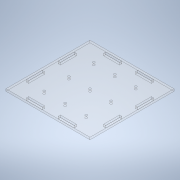
# Autodesk Inventor part: Box top
Saved by Autodesk Inventor 2021 (Build 250183000, 183)
## iProperties
Created: 2019-12-19
Part Number: Box top
Material: PMMA Plastic
Document SubType Name: Modeling
Designer: jstr255
Density: 1.188 g/cm^3
Appearance: Polycarbonate - Clear
Mass: 42.6667 g
Surface Area: 267.032 cm^2
Volume: 35.9147 cm^3
Author: jstr255
Autodesk Inventor part; units mm, degrees
ref_plane "YZ Plane" through (0, 0, 0) normal (1, 0, 0) x (0, 1, 0)
ref_plane "XZ Plane" through (0, 0, 0) normal (0, 1, 0) x (-1, 0, 0)
ref_plane "XY Plane" through (0, 0, 0) normal (0, 0, 1) x (1, 0, 0)
sketch "Sketch1" plane through (0, 0, 0) normal (0, 1, 0) x (-1, 0, 0)
  line L0 (21.2, 0) -> (21.2, -3)
  line L1 (42.4, 0) -> (42.4, -3)
  line L2 (63.6, 0) -> (63.6, -3)
  line L3 (84.8, 0) -> (84.8, -3)
  line L4 (84.8, 0) -> (106, 0)
  line L5 (0, 0) -> (21.2, 0)
  line L6 (42.4, 0) -> (63.6, 0)
  line L7 (21.2, -3) -> (42.4, -3)
  line L8 (63.6, -3) -> (84.8, -3)
  line L9 (106, -21.2) -> (103, -21.2)
  line L10 (106, -42.4) -> (103, -42.4)
  line L11 (106, -63.6) -> (103, -63.6)
  line L12 (106, -84.8) -> (103, -84.8)
  line L13 (106, -84.8) -> (106, -106)
  line L14 (103, -21.2) -> (103, -42.4)
  line L15 (103, -63.6) -> (103, -84.8)
  line L16 (106, 0) -> (106, -21.2)
  line L17 (106, -42.4) -> (106, -63.6)
  line L18 (0, -21.2) -> (3, -21.2)
  line L19 (0, -42.4) -> (3, -42.4)
  line L20 (0, -63.6) -> (3, -63.6)
  line L21 (0, -84.8) -> (3, -84.8)
  line L22 (0, -21.2) -> (0, 0)
  line L23 (3, -84.8) -> (3, -63.6)
  line L24 (3, -42.4) -> (3, -21.2)
  line L25 (0, -106) -> (0, -84.8)
  line L26 (0, -63.6) -> (0, -42.4)
  line L27 (21.2, -106) -> (21.2, -103)
  line L28 (42.4, -106) -> (42.4, -103)
  line L29 (63.6, -106) -> (63.6, -103)
  line L30 (84.8, -106) -> (84.8, -103)
  line L31 (21.2, -106) -> (0, -106)
  line L32 (84.8, -103) -> (63.6, -103)
  line L33 (42.4, -103) -> (21.2, -103)
  line L34 (106, -106) -> (84.8, -106)
  line L35 (63.6, -106) -> (42.4, -106)
  dimension "d0" = 106
  dimension "d1" = 106
  constraints: 72 end point, 45 perpendicular, 26 parallel, 5 horizontal
  measures "d0" distance of L13.end L25.start
  measures "d1" distance of L4.end L13.end
extrude "Extrusion1" add sketch "Sketch1" along normal blind 3
sketch "Sketch2" plane through (0, 3, 0) normal (0, 1, 0) x (1, 0, 0)
  circle A0 centre (-25, 20) radius 0.5
  circle A1 centre (-53, 20) radius 0.5
  circle A2 centre (-81, 20) radius 0.5
  circle A3 centre (-81, 53) radius 0.5
  circle A4 centre (-81, 86) radius 0.5
  circle A5 centre (-53, 53) radius 0.5
  circle A6 centre (-53, 86) radius 0.5
  circle A7 centre (-25, 53) radius 0.5
  circle A8 centre (-25, 86) radius 0.5
  point P0 (0, 0)
  dimension "d6" = 1
  dimension "d7" = 1
  dimension "d8" = 1
  dimension "d9" = 1
  dimension "d10" = 1
  dimension "d11" = 1
  dimension "d12" = 1
  dimension "d13" = 1
  dimension "d14" = 1
  constraints: 9 centre point
  measures "d6" diameter of A0
  measures "d7" diameter of A1
  measures "d8" diameter of A2
  measures "d9" diameter of A3
  measures "d10" diameter of A4
  measures "d11" diameter of A5
  measures "d12" diameter of A6
  measures "d13" diameter of A7
  measures "d14" diameter of A8
hole "Hole1" at (-81, 3, -20) direction (0, -1, 0) diameter 3 end through all
sketch "Sketch3" plane through (0, 3, 0) normal (0, 1, 0) x (1, 0, 0)
  line L0 (-21.2, 0) -> (0, 0) projected
  line L1 (0, 0) -> (-106, 0)
  line L2 (-106, 0) -> (-106, 106)
  line L3 (-106, 106) -> (0, 106)
  line L4 (0, 106) -> (0, 0)
  line L5 (3, -3) -> (-109, -3)
  line L6 (-109, -3) -> (-109, 109)
  line L7 (-109, 109) -> (3, 109)
  line L8 (3, 109) -> (3, -3)
  dimension "d22" = 112
  dimension "d23" = 112
  constraints: 16 end point, 4 parallel, 2 horizontal, 2 perpendicular
  measures "d22" distance of L6.end L7.end
  measures "d23" distance of L5.end L6.end
extrude "Extrusion2" add sketch "Sketch3" against normal blind 3
sketch "Sketch5" plane through (0, 0, 0) normal (0, -1, 0) x (1, 0, 0)
  circle A0 centre (-25, -20) radius 1.5
  point P0 (0, 0)
  dimension "d26" = 3
  constraints: 1 centre point
  measures "d26" diameter of A0
hole "Hole2" at (-25, 0, -20) direction (0, 1, 0) diameter 3 end through all
sketch "Sketch6" plane through (0, 0, 0) normal (0, -1, 0) x (1, 0, 0)
  circle A0 centre (-25, -53) radius 1.5
  point P0 (0, 0)
  dimension "d34" = 3
  constraints: 1 centre point
  measures "d34" diameter of A0
hole "Hole3" at (-25, 0, -53) direction (0, 1, 0) diameter 3 end through all
sketch "Sketch7" plane through (0, 0, 0) normal (0, -1, 0) x (1, 0, 0)
  circle A0 centre (-53, -20) radius 1.5
  point P0 (0, 0)
  dimension "d42" = 3
  constraints: 1 centre point
  measures "d42" diameter of A0
hole "Hole4" at (-53, 0, -20) direction (0, 1, 0) diameter 3 end through all
sketch "Sketch8" plane through (0, 0, 0) normal (0, -1, 0) x (1, 0, 0)
  circle A0 centre (-53, -53) radius 1.5
  point P0 (0, 0)
  dimension "d50" = 3
  constraints: 1 centre point
  measures "d50" diameter of A0
hole "Hole5" at (-53, 0, -53) direction (0, 1, 0) diameter 3 end through all
sketch "Sketch9" plane through (0, 0, 0) normal (0, -1, 0) x (1, 0, 0)
  circle A0 centre (-25, -86) radius 1.5
  point P0 (0, 0)
  dimension "d58" = 3
  constraints: 1 centre point
  measures "d58" diameter of A0
hole "Hole6" at (-25, 0, -86) direction (0, 1, 0) diameter 3 end through all
sketch "Sketch10" plane through (0, 0, 0) normal (0, -1, 0) x (1, 0, 0)
  circle A0 centre (-53, -86) radius 1.5
  point P0 (0, 0)
  dimension "d66" = 3
  constraints: 1 centre point
  measures "d66" diameter of A0
hole "Hole7" at (-53, 0, -86) direction (0, 1, 0) diameter 3 end through all
sketch "Sketch11" plane through (0, 0, 0) normal (0, -1, 0) x (1, 0, 0)
  circle A0 centre (-81, -53) radius 1.5
  point P0 (0, 0)
  dimension "d74" = 3
  constraints: 1 centre point
  measures "d74" diameter of A0
hole "Hole8" at (-81, 0, -53) direction (0, 1, 0) diameter 3 end through all
sketch "Sketch12" plane through (0, 0, 0) normal (0, -1, 0) x (1, 0, 0)
  circle A0 centre (-81, -86) radius 1.5
  point P0 (0, 0)
  dimension "d82" = 3
  constraints: 1 centre point
  measures "d82" diameter of A0
hole "Hole9" at (-81, 0, -86) direction (0, 1, 0) diameter 3 end through all
body "Solid1"
